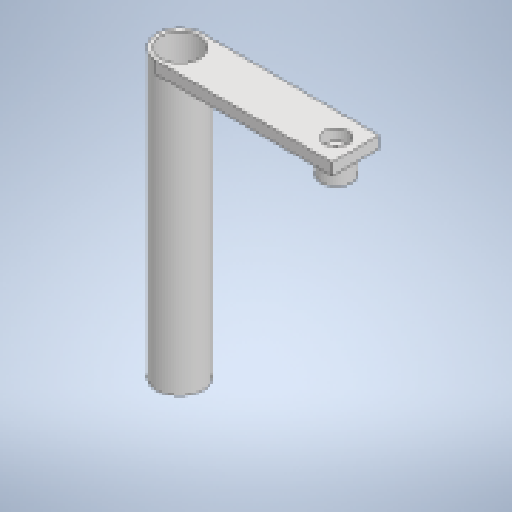
# Autodesk Inventor part: pole-1
Saved by Autodesk Inventor 2025 (Build 290162000, 162)
## iProperties
Created: 2026-01-27
Part Number: pole-1
Material: 一般
Document SubType Name: Modeling
Designer: mahhy
Density: 1 g/cm^3
Appearance: 既定
Author: mahhy
Autodesk Inventor part; units mm, degrees
ref_plane "YZ Plane" through (0, 0, 0) normal (1, 0, 0) x (0, 1, 0)
ref_plane "XZ Plane" through (0, 0, 0) normal (0, 1, 0) x (-1, 0, 0)
ref_plane "XY Plane" through (0, 0, 0) normal (0, 0, 1) x (1, 0, 0)
sketch "軸スケッチ" plane through (0, 0, 0) normal (0, 1, 0) x (-1, 0, 0)
  circle A0 centre (0, 0) radius 6
  circle A1 centre (0, 0) radius 5
  dimension "d0" = 12
  dimension "d1" = 10
  constraints: 2 centre point, 2 coincident
  measures "d0" diameter of A0
  measures "d1" diameter of A1
extrude "軸" add sketch "軸スケッチ" along normal blind 73
sketch "アームスケッチ" plane through (0, 73, 0) normal (0, 1, 0) x (1, 0, 0)
  circle A0 centre (0, 0) radius 6 projected
  line L0 (0, -6) -> (45, -6)
  line L1 (45, -6) -> (45, 6)
  line L2 (45, 6) -> (0, 6)
  line L3 (0, 6) -> (0, -6)
  circle A1 centre (40, 0) radius 1.6
  point P0 (45, 0)
  dimension "d9" = 45
  dimension "d10" = 12
  dimension "d18" = 3.2
  dimension "d19" = 5
  constraints: 8 end point, 2 parallel, 2 point on circle, 1 centre point, 1 horizontal, 1 horizontal alignment, 1 midpoint, 1 perpendicular
  measures "d9" distance of L2.end L1.end
  measures "d10" distance of L1.end L0.end
  measures "d18" diameter of A1
  measures "d19" distance from line of L1 A1.centre
extrude "アーム" add sketch "アームスケッチ" against normal blind 3 contours A0 L2 L1 L0
sketch "接合部スケッチ" plane through (0, 70, 0) normal (0, -1, 0) x (1, 0, 0)
  circle A0 centre (40, 0) radius 4
  line L0 (45, -6) -> (45, 6) projected
  circle A1 centre (40, 0) radius 1.6 projected
  point P0 (0, 0)
  point P1 (45, 0)
  dimension "d13" = 8
  dimension "d14" = 5
  dimension "d15" = 40
  constraints: 1 centre point, 1 horizontal alignment, 1 midpoint
  measures "d13" diameter of A0
  measures "d14" distance from line of L0 A0.centre
  measures "d15" distance of point (0, 0) A0.centre
extrude "接合部" add sketch "接合部スケッチ" along normal blind 5
sketch "スケッチ4" plane through (0, 73, 0) normal (0, 1, 0) x (1, 0, 0)
  circle A0 centre (40, 0) radius 1.6 projected
  circle A1 centre (40, 0) radius 3
  point P0 (0, 0)
  dimension "d20" = 6
  constraints: 1 centre point, 1 coincident
  measures "d20" diameter of A1
extrude "ねじ頭" cut sketch "スケッチ4" against normal blind 3
